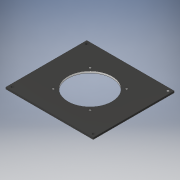
# Autodesk Inventor part: Base Cover Left
Saved by Autodesk Inventor 2019 (Build 230136000, 136)
## iProperties
Created: 2018-11-05
Part Number: Base Cover Left
Material: Generic
Document SubType Name: Modeling
Designer: Keith
Density: 1 g/cm^3
Appearance: Default
Author: Keith
## iProperties of the stored document Base Cover Left 60mm Fan_3DPrint.ipt
Created: 2019-02-26
Part Number: Base Cover Left 60mm Fan_3DPrint
Material: Generic
Document SubType Name: Modeling
Designer: Keith
Density: 1 g/cm^3
Appearance: Default
Author: Keith
Autodesk Inventor part; units mm, degrees
ref_plane "YZ Plane" through (0, 0, 0) normal (1, 0, 0) x (0, 1, 0)
ref_plane "XZ Plane" through (0, 0, 0) normal (0, 1, 0) x (-1, 0, 0)
sketch "Sketch1" plane through (0, 0, 0) normal (0, 1, 0) x (-1, 0, 0)
  line L0 (0, 0) -> (119, 0)
  line L1 (119, 0) -> (119, -110.2)
  line L2 (119, -110.2) -> (0, -110.2)
  line L3 (0, -110.2) -> (0, 0)
  dimension "d0" = 119
  dimension "d1" = 110.2
  constraints: 8 end point, 2 parallel, 1 horizontal, 1 perpendicular
  measures "d0" distance of L1.end L2.end
  measures "d1" distance of L0.end L1.end
extrude "Extrusion1" add sketch "Sketch1" along normal blind 2.5
sketch "Sketch2" plane through (0, 2.5, 0) normal (0, 1, 0) x (1, 0, 0)
  line L0 (-119, 0) -> (0, 0) projected
  line L1 (0, 0) -> (0, 110.2) projected
  line L2 (0, 110.2) -> (-119, 110.2) projected
  line L3 (-119, 110.2) -> (-119, 0) projected
  circle A0 centre (-114.875, 4.375) radius 1.55
  circle A1 centre (-11.5301, 10.067) radius 1.55
  circle A2 centre (-11.5301, 99.7072) radius 1.55
  circle A3 centre (-114.875, 105.95) radius 1.55
  dimension "d4" = 3.1
  dimension "d5" = 3.1
  dimension "d6" = 3.1
  dimension "d7" = 3.1
  dimension "d8" = 4.375
  dimension "d9" = 4.125
  dimension "d10" = 4.25
  dimension "d11" = 4.125
  constraints: 4 centre point
  measures "d4" diameter of A0
  measures "d5" diameter of A1
  measures "d6" diameter of A2
  measures "d7" diameter of A3
  measures "d8" distance from line of L0 A0.centre
  measures "d9" distance from line of L3 A0.centre
  measures "d10" distance from line of L2 A3.centre
  measures "d11" distance from line of L3 A3.centre
extrude "Extrusion2" cut sketch "Sketch2" against normal through all contours A0 | A3
ref_plane "Work Plane1" through (-59.5, 0, 0) normal (1, 0, 0) x (0, 0, -1)
mirror "Mirror1" about plane through (-59.5, 0, 0) normal (1, 0, 0) of "Extrusion2"
sketch "Sketch3" plane through (0, 2.5, 0) normal (0, 1, 0) x (1, 0, 0)
  circle A0 centre (-4.125, 4.375) radius 1.55 projected
  circle A1 centre (-4.125, 105.95) radius 1.55 projected
  circle A2 centre (-114.875, 4.375) radius 1.55 projected
  circle A3 centre (-114.875, 105.95) radius 1.55 projected
  line L0 (-119, 0) -> (0, 0) projected
  line L1 (0, 0) -> (0, 110.2) projected
  line L2 (0, 110.2) -> (-119, 110.2) projected
  line L3 (-119, 110.2) -> (-119, 0) projected
  circle A4 centre (-59.5, 55.1) radius 30
  circle A5 centre (-34.5, 80.1) radius 1.35
  circle A6 centre (-34.5, 30.1) radius 1.35
  circle A7 centre (-84.5, 30.1) radius 1.35
  circle A8 centre (-84.5, 80.1) radius 1.35
  dimension "d26" = 2.7
  dimension "d27" = 2.7
  dimension "d30" = 50
  dimension "d31" = 50
  dimension "d32" = 50
  dimension "d33" = 25
  dimension "d34" = 25
  dimension "d35" = 25
  dimension "d36" = 60
  constraints: 5 centre point
  measures "d26" diameter of A7
  measures "d27" diameter of A8
  measures "d30" distance of A5.centre A8.centre
  measures "d31" distance of A6.centre A7.centre
  measures "d32" distance between centres of A8 A7
  measures "d33" horizontal distance of A8.centre A4.centre
  measures "d34" horizontal distance of A4.centre A5.centre
  measures "d35" horizontal distance of A4.centre A8.centre
  measures "d36" diameter of A4
extrude "Extrusion3" cut sketch "Sketch3" against normal through all contours A4 | A5 | A6 | A7 | A8
body "Solid1"
